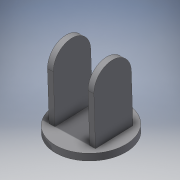
# Autodesk Inventor part: swivel
Saved by Autodesk Inventor 2020 (Build 240168000, 168)
## iProperties
Created: 2020-02-04
Part Number: swivel
Material: Generic
Document SubType Name: Modeling
Designer: Wes
Density: 1 g/cm^3
Appearance: Default
Author: Wes
Autodesk Inventor part; units mm, degrees
ref_plane "YZ Plane" through (0, 0, 0) normal (1, 0, 0) x (0, 1, 0)
ref_plane "XZ Plane" through (0, 0, 0) normal (0, 1, 0) x (-1, 0, 0)
ref_plane "XY Plane" through (0, 0, 0) normal (0, 0, 1) x (1, 0, 0)
sketch "Sketch1 - walls" plane through (0, 0, 0) normal (0, 0, 1) x (1, 0, 0)
  line L0 (0, -9) -> (0, 9) construction
  line L1 (-10, -9) -> (-10, -12)
  line L2 (-10, -12) -> (10, -12)
  line L3 (-10, -9) -> (10, -9)
  line L4 (10, -9) -> (10, -12)
  line L5 (-10, 9) -> (10, 9)
  line L6 (10, 9) -> (10, 12)
  line L7 (10, 12) -> (-10, 12)
  line L8 (-10, 12) -> (-10, 9)
  point P0 (0, 0)
  dimension "d5" = 18
  dimension "d7" = 3
  dimension "d8" = 20
  dimension "d9" = 3
  dimension "d10" = 20
  constraints: 18 end point, 4 perpendicular, 3 horizontal, 2 vertical
  measures "d5" distance of L0.start L0.end
  measures "d7" distance of L1.start L1.end
  measures "d8" distance of L1.end L2.end
  measures "d9" distance of L5.end L6.end
  measures "d10" distance of L6.end L7.end
extrude "Extrusion1" add sketch "Sketch1 - walls" along normal blind 25
sketch "Sketch2 - base" plane through (0, 0, 0) normal (0, 0, -1) x (-1, 0, 0)
  circle A0 centre (0, 0) radius 18.5
  dimension "d13" = 37
  constraints: 1 centre point, 1 coincident
  measures "d13" diameter of A0
sketch "Sketch3 - wall_top1" plane through (-10, 12, 25) normal (0, 1, 0) x (1, 0, 0)
  line L0 (10, 0) -> (10, -10) construction
  line L1 (20, 0) -> (0, 0) projected
  arc A0 (0, 0) -> (20, 0) centre (10, 0) ccw
  point P0 (10, 25)
  dimension "d16" = 10
  constraints: 3 point on circle, 2 end point, 1 centre point
  measures "d16" distance of L0.start L0.end
extrude "Extrusion3" add sketch "Sketch3 - wall_top1" against normal blind 3
sketch "Sketch4 - wall_top2" plane through (-10, -12, 25) normal (0, -1, 0) x (1, 0, 0)
  line L0 (10, 0) -> (10, 10) construction
  line L1 (0, 0) -> (20, 0) projected
  arc A0 (20, 0) -> (0, 0) centre (10, 0) ccw
  dimension "d21" = 10
  constraints: 3 point on circle, 2 end point, 1 centre point, 1 vertical
  measures "d21" distance of L0.start L0.end
extrude "Extrusion4" add sketch "Sketch4 - wall_top2" against normal blind 3
extrude "Extrusion2" add sketch "Sketch2 - base" along normal blind 3.5
body "Solid2"
